tappopannello (Autodesk Fusion 360 design; units mm, degrees)
Autodesk Fusion 360 part; units mm, degrees
sketch "Sketch1" plane through (0, 0, 0) normal (0, 0, 1) x (1, 0, 0)
  line L0 (10, -10) -> (-10, -10)
  line L1 (-10, -10) -> (-10, 10)
  line L2 (-10, 10) -> (10, 10)
  line L3 (10, 10) -> (10, -10)
  line L4 (10, -10) -> (-10, 10) construction
  line L5 (-10, -10) -> (10, 10) construction
  line L6 (11.75, -11.75) -> (-11.75, -11.75)
  line L7 (-11.75, -11.75) -> (-11.75, 11.75)
  line L8 (-11.75, 11.75) -> (11.75, 11.75)
  line L9 (11.75, 11.75) -> (11.75, -11.75)
  line L10 (11.75, -11.75) -> (-11.75, 11.75) construction
  line L11 (-11.75, -11.75) -> (11.75, 11.75) construction
  dimension "d1" = 20
  dimension "d2" = 20
  dimension "d3" = 23.5
  dimension "d4" = 23.5
  constraint horizontal L0
  constraint perpendicular L0 L1
  constraint parallel L0 L2
  constraint parallel L1 L3
  constraint coincident L4 origin
  constraint coincident L5 origin
  constraint horizontal L6
  constraint perpendicular L6 L7
  constraint parallel L6 L8
  constraint parallel L7 L9
  constraint coincident L10 origin
  constraint coincident L11 origin
  measures "d1" distance of L1.end L2.end
  measures "d2" distance of L0.end L1.end
  measures "d3" distance of L7.end L8.end
  measures "d4" distance of L6.end L7.end
extrude "Extrude1" add sketch "Sketch1" along normal blind 15 contours L0 L1 L2 L3 | L6 L7 L8 L9
extrude "Extrude2" cut sketch "Sketch1" along normal blind 12
fillet "Fillet1" radius 1 4 edges at (11.75, 11.75, 13.5) (-11.75, 11.75, 13.5) (11.75, -11.75, 13.5) (-11.75, -11.75, 13.5)
fillet "Fillet2" radius 1 4 edges at (-10, 10, 6) (10, 10, 6) (10, -10, 6) (-10, -10, 6)
fillet "Fillet3" radius 1.2 8 edges at (-11.4571, 11.4571, 15) (-11.75, 0, 15) (-11.4571, -11.4571, 15) (0, -11.75, 15) (11.4571, -11.4571, 15) (11.75, 0, 15) (11.4571, 11.4571, 15) (0, 11.75, 15)
